Autodesk Fusion 360 part; units mm, degrees
(part 2 of 7)
  spline S30 degree 3 poles (-152.5, -27.3069) (-152.0881, -26.4817) (-151.6514, -25.2172) (-151.2668, -23.9183) (-150.7129, -22.0478) (-150.237, -20.0931) (-149.6002, -18.3797) (-148.9085, -16.5186) (-147.986, -14.8851) (-146.6355, -13.7409) (-146.4823, -13.6111) (-146.3242, -13.4878) (-146.1613, -13.3717) (-145.7742, -13.0956) (-145.3871, -12.8196) (-145, -12.5435) knots -0.398144 -0.398144 -0.398144 -0.398144 -0.30293 -0.30293 -0.30293 -0.165823 -0.165823 -0.165823 -0.016893 -0.016893 -0.016893 0 0 0 0.056001 0.056001 0.056001 0.056001
  spline S31 degree 3 poles (-145, -12.5435) (-144.6129, -12.8196) (-144.2258, -13.0956) (-143.8387, -13.3717) (-142.4048, -14.3943) (-141.3881, -15.9477) (-140.6468, -17.7479) (-139.9554, -19.4267) (-139.4675, -21.3627) (-138.9195, -23.2775) (-138.5808, -24.4611) (-138.2149, -25.6362) (-137.8326, -26.5675) (-137.7208, -26.8397) (-137.6088, -27.0889) (-137.5, -27.3069) knots -1.056001 -1.056001 -1.056001 -1.056001 -1 -1 -1 -0.851292 -0.851292 -0.851292 -0.71262 -0.71262 -0.71262 -0.626906 -0.626906 -0.626906 -0.601856 -0.601856 -0.601856 -0.601856
  spline S32 degree 3 poles (-137.5, -27.3069) (-137.0881, -26.4817) (-136.6514, -25.2172) (-136.2668, -23.9183) (-135.7129, -22.0478) (-135.237, -20.0931) (-134.6002, -18.3797) (-133.9085, -16.5186) (-132.986, -14.8851) (-131.6355, -13.7409) (-131.4823, -13.6111) (-131.3242, -13.4878) (-131.1613, -13.3717) (-130.7742, -13.0956) (-130.3871, -12.8196) (-130, -12.5435) knots -0.398144 -0.398144 -0.398144 -0.398144 -0.30293 -0.30293 -0.30293 -0.165823 -0.165823 -0.165823 -0.016893 -0.016893 -0.016893 0 0 0 0.056001 0.056001 0.056001 0.056001
  spline S33 degree 3 poles (-130, -12.5435) (-129.6129, -12.8196) (-129.2258, -13.0956) (-128.8387, -13.3717) (-127.4048, -14.3943) (-126.3881, -15.9477) (-125.6468, -17.7479) (-124.9554, -19.4267) (-124.4675, -21.3627) (-123.9195, -23.2775) (-123.5808, -24.4611) (-123.2149, -25.6362) (-122.8326, -26.5675) (-122.7208, -26.8397) (-122.6088, -27.0889) (-122.5, -27.3069) knots -1.056001 -1.056001 -1.056001 -1.056001 -1 -1 -1 -0.851292 -0.851292 -0.851292 -0.71262 -0.71262 -0.71262 -0.626906 -0.626906 -0.626906 -0.601856 -0.601856 -0.601856 -0.601856
  spline S34 degree 3 poles (-122.5, -27.3069) (-122.0881, -26.4817) (-121.6514, -25.2172) (-121.2668, -23.9183) (-120.7129, -22.0478) (-120.237, -20.0931) (-119.6002, -18.3797) (-118.9085, -16.5186) (-117.986, -14.8851) (-116.6355, -13.7409) (-116.4823, -13.6111) (-116.3242, -13.4878) (-116.1613, -13.3717) (-115.7742, -13.0956) (-115.3871, -12.8196) (-115, -12.5435) knots -0.398144 -0.398144 -0.398144 -0.398144 -0.30293 -0.30293 -0.30293 -0.165823 -0.165823 -0.165823 -0.016893 -0.016893 -0.016893 0 0 0 0.056001 0.056001 0.056001 0.056001
  spline S35 degree 3 poles (-115, -12.5435) (-114.6129, -12.8196) (-114.2258, -13.0956) (-113.8387, -13.3717) (-112.4048, -14.3943) (-111.3881, -15.9477) (-110.6468, -17.7479) (-109.9554, -19.4267) (-109.4675, -21.3627) (-108.9195, -23.2775) (-108.5808, -24.4611) (-108.2149, -25.6362) (-107.8326, -26.5675) (-107.7208, -26.8397) (-107.6088, -27.0889) (-107.5, -27.3069) knots -1.056001 -1.056001 -1.056001 -1.056001 -1 -1 -1 -0.851292 -0.851292 -0.851292 -0.71262 -0.71262 -0.71262 -0.626906 -0.626906 -0.626906 -0.601856 -0.601856 -0.601856 -0.601856
  spline S36 degree 3 poles (-107.5, -27.3069) (-107.0881, -26.4817) (-106.6514, -25.2172) (-106.2668, -23.9183) (-105.7129, -22.0478) (-105.237, -20.0931) (-104.6002, -18.3797) (-103.9085, -16.5186) (-102.986, -14.8851) (-101.6355, -13.7409) (-101.4823, -13.6111) (-101.3242, -13.4878) (-101.1613, -13.3717) (-100.7742, -13.0956) (-100.3871, -12.8196) (-100, -12.5435) knots -0.398144 -0.398144 -0.398144 -0.398144 -0.30293 -0.30293 -0.30293 -0.165823 -0.165823 -0.165823 -0.016893 -0.016893 -0.016893 0 0 0 0.056001 0.056001 0.056001 0.056001
  spline S37 degree 3 poles (-100, -12.5435) (-99.6129, -12.8196) (-99.2258, -13.0956) (-98.8387, -13.3717) (-97.4048, -14.3943) (-96.3881, -15.9477) (-95.6468, -17.7479) (-94.9554, -19.4267) (-94.4675, -21.3627) (-93.9195, -23.2775) (-93.5808, -24.4611) (-93.2149, -25.6362) (-92.8326, -26.5675) (-92.7208, -26.8397) (-92.6088, -27.0889) (-92.5, -27.3069) knots -1.056001 -1.056001 -1.056001 -1.056001 -1 -1 -1 -0.851292 -0.851292 -0.851292 -0.71262 -0.71262 -0.71262 -0.626906 -0.626906 -0.626906 -0.601856 -0.601856 -0.601856 -0.601856
  spline S38 degree 3 poles (-92.5, -27.3069) (-92.0881, -26.4817) (-91.6514, -25.2172) (-91.2668, -23.9183) (-90.7129, -22.0478) (-90.237, -20.0931) (-89.6002, -18.3797) (-88.9085, -16.5186) (-87.986, -14.8851) (-86.6355, -13.7409) (-86.4823, -13.6111) (-86.3242, -13.4878) (-86.1613, -13.3717) (-85.7742, -13.0956) (-85.3871, -12.8196) (-85, -12.5435) knots -0.398144 -0.398144 -0.398144 -0.398144 -0.30293 -0.30293 -0.30293 -0.165823 -0.165823 -0.165823 -0.016893 -0.016893 -0.016893 0 0 0 0.056001 0.056001 0.056001 0.056001
  spline S39 degree 3 poles (-85, -12.5435) (-84.6129, -12.8196) (-84.2258, -13.0956) (-83.8387, -13.3717) (-82.4048, -14.3943) (-81.3881, -15.9477) (-80.6468, -17.7479) (-79.9554, -19.4267) (-79.4675, -21.3627) (-78.9195, -23.2775) (-78.5808, -24.4611) (-78.2149, -25.6362) (-77.8326, -26.5675) (-77.7208, -26.8397) (-77.6088, -27.0889) (-77.5, -27.3069) knots -1.056001 -1.056001 -1.056001 -1.056001 -1 -1 -1 -0.851292 -0.851292 -0.851292 -0.71262 -0.71262 -0.71262 -0.626906 -0.626906 -0.626906 -0.601856 -0.601856 -0.601856 -0.601856
  spline S40 degree 3 poles (-77.5, -27.3069) (-77.0881, -26.4817) (-76.6514, -25.2172) (-76.2668, -23.9183) (-75.7129, -22.0478) (-75.237, -20.0931) (-74.6002, -18.3797) (-73.9085, -16.5186) (-72.986, -14.8851) (-71.6355, -13.7409) (-71.4823, -13.6111) (-71.3242, -13.4878) (-71.1613, -13.3717) (-70.7742, -13.0956) (-70.3871, -12.8196) (-70, -12.5435) knots -0.398144 -0.398144 -0.398144 -0.398144 -0.30293 -0.30293 -0.30293 -0.165823 -0.165823 -0.165823 -0.016893 -0.016893 -0.016893 0 0 0 0.056001 0.056001 0.056001 0.056001
  spline S41 degree 3 poles (-70, -12.5435) (-69.6129, -12.8196) (-69.2258, -13.0956) (-68.8387, -13.3717) (-67.4048, -14.3943) (-66.3881, -15.9477) (-65.6468, -17.7479) (-64.9554, -19.4267) (-64.4675, -21.3627) (-63.9195, -23.2775) (-63.5808, -24.4611) (-63.2149, -25.6362) (-62.8326, -26.5675) (-62.7208, -26.8397) (-62.6088, -27.0889) (-62.5, -27.3069) knots -1.056001 -1.056001 -1.056001 -1.056001 -1 -1 -1 -0.851292 -0.851292 -0.851292 -0.71262 -0.71262 -0.71262 -0.626906 -0.626906 -0.626906 -0.601856 -0.601856 -0.601856 -0.601856
  spline S42 degree 3 poles (-62.5, -27.3069) (-62.0881, -26.4817) (-61.6514, -25.2172) (-61.2668, -23.9183) (-60.7129, -22.0478) (-60.237, -20.0931) (-59.6002, -18.3797) (-58.9085, -16.5186) (-57.986, -14.8851) (-56.6355, -13.7409) (-56.4823, -13.6111) (-56.3242, -13.4878) (-56.1613, -13.3717) (-55.7742, -13.0956) (-55.3871, -12.8196) (-55, -12.5435) knots -0.398144 -0.398144 -0.398144 -0.398144 -0.30293 -0.30293 -0.30293 -0.165823 -0.165823 -0.165823 -0.016893 -0.016893 -0.016893 0 0 0 0.056001 0.056001 0.056001 0.056001
  spline S43 degree 3 poles (-55, -12.5435) (-54.6129, -12.8196) (-54.2258, -13.0956) (-53.8387, -13.3717) (-52.4048, -14.3943) (-51.3881, -15.9477) (-50.6468, -17.7479) (-49.9554, -19.4267) (-49.4675, -21.3627) (-48.9195, -23.2775) (-48.5808, -24.4611) (-48.2149, -25.6362) (-47.8326, -26.5675) (-47.7208, -26.8397) (-47.6088, -27.0889) (-47.5, -27.3069) knots -1.056001 -1.056001 -1.056001 -1.056001 -1 -1 -1 -0.851292 -0.851292 -0.851292 -0.71262 -0.71262 -0.71262 -0.626906 -0.626906 -0.626906 -0.601856 -0.601856 -0.601856 -0.601856
  spline S44 degree 3 poles (-47.5, -27.3069) (-47.0881, -26.4817) (-46.6514, -25.2172) (-46.2668, -23.9183) (-45.7129, -22.0478) (-45.237, -20.0931) (-44.6002, -18.3797) (-43.9085, -16.5186) (-42.986, -14.8851) (-41.6355, -13.7409) (-41.4823, -13.6111) (-41.3242, -13.4878) (-41.1613, -13.3717) (-40.7742, -13.0956) (-40.3871, -12.8196) (-40, -12.5435) knots -0.398144 -0.398144 -0.398144 -0.398144 -0.30293 -0.30293 -0.30293 -0.165823 -0.165823 -0.165823 -0.016893 -0.016893 -0.016893 0 0 0 0.056001 0.056001 0.056001 0.056001
  spline S45 degree 3 poles (-40, -12.5435) (-39.6129, -12.8196) (-39.2258, -13.0956) (-38.8387, -13.3717) (-37.4048, -14.3943) (-36.3881, -15.9477) (-35.6468, -17.7479) (-34.9554, -19.4267) (-34.4675, -21.3627) (-33.9195, -23.2775) (-33.5808, -24.4611) (-33.2149, -25.6362) (-32.8326, -26.5675) (-32.7208, -26.8397) (-32.6088, -27.0889) (-32.5, -27.3069) knots -1.056001 -1.056001 -1.056001 -1.056001 -1 -1 -1 -0.851292 -0.851292 -0.851292 -0.71262 -0.71262 -0.71262 -0.626906 -0.626906 -0.626906 -0.601856 -0.601856 -0.601856 -0.601856
  spline S46 degree 3 poles (-32.5, -27.3069) (-32.0881, -26.4817) (-31.6514, -25.2172) (-31.2668, -23.9183) (-30.7129, -22.0478) (-30.237, -20.0931) (-29.6002, -18.3797) (-28.9085, -16.5186) (-27.986, -14.8851) (-26.6355, -13.7409) (-26.4823, -13.6111) (-26.3242, -13.4878) (-26.1613, -13.3717) (-25.7742, -13.0956) (-25.3871, -12.8196) (-25, -12.5435) knots -0.398144 -0.398144 -0.398144 -0.398144 -0.30293 -0.30293 -0.30293 -0.165823 -0.165823 -0.165823 -0.016893 -0.016893 -0.016893 0 0 0 0.056001 0.056001 0.056001 0.056001
  arc A14 (-250, -12.5435) -> (-250, -3) centre (-250, -7.7718) ccw
  arc A15 (-25, -3) -> (-25, -12.5435) centre (-25, -7.7718) ccw
  constraint tangent L29 A14
  constraint coincident L29 A14.end
  constraint tangent L29 A15
  constraint coincident L29 A15.start
sketch "スケッチ6" plane through (0, 0, 2) normal (0, 0, 1) x (-1, 0, 0)
  spline S0 degree 3 poles (-242.5, -27.3069) (-242.6088, -27.0889) (-242.7208, -26.8397) (-242.8326, -26.5675) (-243.2149, -25.6362) (-243.5808, -24.4611) (-243.9195, -23.2775) (-244.4675, -21.3627) (-244.9554, -19.4267) (-245.6468, -17.7479) (-246.3881, -15.9477) (-247.4048, -14.3943) (-248.8387, -13.3717) (-249.2258, -13.0956) (-249.6129, -12.8196) (-250, -12.5435) knots 0.601856 0.601856 0.601856 0.601856 0.626906 0.626906 0.626906 0.71262 0.71262 0.71262 0.851292 0.851292 0.851292 1 1 1 1.056001 1.056001 1.056001 1.056001
  spline S1 degree 3 poles (-235, -12.5435) (-235.3871, -12.8196) (-235.7742, -13.0956) (-236.1613, -13.3717) (-236.3242, -13.4878) (-236.4823, -13.6111) (-236.6355, -13.7409) (-237.986, -14.8851) (-238.9085, -16.5186) (-239.6002, -18.3797) (-240.237, -20.0931) (-240.7129, -22.0478) (-241.2668, -23.9183) (-241.6514, -25.2172) (-242.0881, -26.4817) (-242.5, -27.3069) knots -0.056001 -0.056001 -0.056001 -0.056001 0 0 0 0.016893 0.016893 0.016893 0.165823 0.165823 0.165823 0.30293 0.30293 0.30293 0.398144 0.398144 0.398144 0.398144
  spline S2 degree 3 poles (-227.5, -27.3069) (-227.6088, -27.0889) (-227.7208, -26.8397) (-227.8326, -26.5675) (-228.2149, -25.6362) (-228.5808, -24.4611) (-228.9195, -23.2775) (-229.4675, -21.3627) (-229.9554, -19.4267) (-230.6468, -17.7479) (-231.3881, -15.9477) (-232.4048, -14.3943) (-233.8387, -13.3717) (-234.2258, -13.0956) (-234.6129, -12.8196) (-235, -12.5435) knots 0.601856 0.601856 0.601856 0.601856 0.626906 0.626906 0.626906 0.71262 0.71262 0.71262 0.851292 0.851292 0.851292 1 1 1 1.056001 1.056001 1.056001 1.056001
  spline S3 degree 3 poles (-220, -12.5435) (-220.3871, -12.8196) (-220.7742, -13.0956) (-221.1613, -13.3717) (-221.3242, -13.4878) (-221.4823, -13.6111) (-221.6355, -13.7409) (-222.986, -14.8851) (-223.9085, -16.5186) (-224.6002, -18.3797) (-225.237, -20.0931) (-225.7129, -22.0478) (-226.2668, -23.9183) (-226.6514, -25.2172) (-227.0881, -26.4817) (-227.5, -27.3069) knots -0.056001 -0.056001 -0.056001 -0.056001 0 0 0 0.016893 0.016893 0.016893 0.165823 0.165823 0.165823 0.30293 0.30293 0.30293 0.398144 0.398144 0.398144 0.398144
  spline S4 degree 3 poles (-212.5, -27.3069) (-212.6088, -27.0889) (-212.7208, -26.8397) (-212.8326, -26.5675) (-213.2149, -25.6362) (-213.5808, -24.4611) (-213.9195, -23.2775) (-214.4675, -21.3627) (-214.9554, -19.4267) (-215.6468, -17.7479) (-216.3881, -15.9477) (-217.4048, -14.3943) (-218.8387, -13.3717) (-219.2258, -13.0956) (-219.6129, -12.8196) (-220, -12.5435) knots 0.601856 0.601856 0.601856 0.601856 0.626906 0.626906 0.626906 0.71262 0.71262 0.71262 0.851292 0.851292 0.851292 1 1 1 1.056001 1.056001 1.056001 1.056001
  spline S5 degree 3 poles (-205, -12.5435) (-205.3871, -12.8196) (-205.7742, -13.0956) (-206.1613, -13.3717) (-206.3242, -13.4878) (-206.4823, -13.6111) (-206.6355, -13.7409) (-207.986, -14.8851) (-208.9085, -16.5186) (-209.6002, -18.3797) (-210.237, -20.0931) (-210.7129, -22.0478) (-211.2668, -23.9183) (-211.6514, -25.2172) (-212.0881, -26.4817) (-212.5, -27.3069) knots -0.056001 -0.056001 -0.056001 -0.056001 0 0 0 0.016893 0.016893 0.016893 0.165823 0.165823 0.165823 0.30293 0.30293 0.30293 0.398144 0.398144 0.398144 0.398144
  spline S6 degree 3 poles (-197.5, -27.3069) (-197.6088, -27.0889) (-197.7208, -26.8397) (-197.8326, -26.5675) (-198.2149, -25.6362) (-198.5808, -24.4611) (-198.9195, -23.2775) (-199.4675, -21.3627) (-199.9554, -19.4267) (-200.6468, -17.7479) (-201.3881, -15.9477) (-202.4048, -14.3943) (-203.8387, -13.3717) (-204.2258, -13.0956) (-204.6129, -12.8196) (-205, -12.5435) knots 0.601856 0.601856 0.601856 0.601856 0.626906 0.626906 0.626906 0.71262 0.71262 0.71262 0.851292 0.851292 0.851292 1 1 1 1.056001 1.056001 1.056001 1.056001
  spline S7 degree 3 poles (-190, -12.5435) (-190.3871, -12.8196) (-190.7742, -13.0956) (-191.1613, -13.3717) (-191.3242, -13.4878) (-191.4823, -13.6111) (-191.6355, -13.7409) (-192.986, -14.8851) (-193.9085, -16.5186) (-194.6002, -18.3797) (-195.237, -20.0931) (-195.7129, -22.0478) (-196.2668, -23.9183) (-196.6514, -25.2172) (-197.0881, -26.4817) (-197.5, -27.3069) knots -0.056001 -0.056001 -0.056001 -0.056001 0 0 0 0.016893 0.016893 0.016893 0.165823 0.165823 0.165823 0.30293 0.30293 0.30293 0.398144 0.398144 0.398144 0.398144
  spline S8 degree 3 poles (-182.5, -27.3069) (-182.6088, -27.0889) (-182.7208, -26.8397) (-182.8326, -26.5675) (-183.2149, -25.6362) (-183.5808, -24.4611) (-183.9195, -23.2775) (-184.4675, -21.3627) (-184.9554, -19.4267) (-185.6468, -17.7479) (-186.3881, -15.9477) (-187.4048, -14.3943) (-188.8387, -13.3717) (-189.2258, -13.0956) (-189.6129, -12.8196) (-190, -12.5435) knots 0.601856 0.601856 0.601856 0.601856 0.626906 0.626906 0.626906 0.71262 0.71262 0.71262 0.851292 0.851292 0.851292 1 1 1 1.056001 1.056001 1.056001 1.056001
  spline S9 degree 3 poles (-175, -12.5435) (-175.3871, -12.8196) (-175.7742, -13.0956) (-176.1613, -13.3717) (-176.3242, -13.4878) (-176.4823, -13.6111) (-176.6355, -13.7409) (-177.986, -14.8851) (-178.9085, -16.5186) (-179.6002, -18.3797) (-180.237, -20.0931) (-180.7129, -22.0478) (-181.2668, -23.9183) (-181.6514, -25.2172) (-182.0881, -26.4817) (-182.5, -27.3069) knots -0.056001 -0.056001 -0.056001 -0.056001 0 0 0 0.016893 0.016893 0.016893 0.165823 0.165823 0.165823 0.30293 0.30293 0.30293 0.398144 0.398144 0.398144 0.398144
  spline S10 degree 3 poles (-167.5, -27.3069) (-167.6088, -27.0889) (-167.7208, -26.8397) (-167.8326, -26.5675) (-168.2149, -25.6362) (-168.5808, -24.4611) (-168.9195, -23.2775) (-169.4675, -21.3627) (-169.9554, -19.4267) (-170.6468, -17.7479) (-171.3881, -15.9477) (-172.4048, -14.3943) (-173.8387, -13.3717) (-174.2258, -13.0956) (-174.6129, -12.8196) (-175, -12.5435) knots 0.601856 0.601856 0.601856 0.601856 0.626906 0.626906 0.626906 0.71262 0.71262 0.71262 0.851292 0.851292 0.851292 1 1 1 1.056001 1.056001 1.056001 1.056001
  spline S11 degree 3 poles (-160, -12.5435) (-160.3871, -12.8196) (-160.7742, -13.0956) (-161.1613, -13.3717) (-161.3242, -13.4878) (-161.4823, -13.6111) (-161.6355, -13.7409) (-162.986, -14.8851) (-163.9085, -16.5186) (-164.6002, -18.3797) (-165.237, -20.0931) (-165.7129, -22.0478) (-166.2668, -23.9183) (-166.6514, -25.2172) (-167.0881, -26.4817) (-167.5, -27.3069) knots -0.056001 -0.056001 -0.056001 -0.056001 0 0 0 0.016893 0.016893 0.016893 0.165823 0.165823 0.165823 0.30293 0.30293 0.30293 0.398144 0.398144 0.398144 0.398144
  spline S12 degree 3 poles (-152.5, -27.3069) (-152.6088, -27.0889) (-152.7208, -26.8397) (-152.8326, -26.5675) (-153.2149, -25.6362) (-153.5808, -24.4611) (-153.9195, -23.2775) (-154.4675, -21.3627) (-154.9554, -19.4267) (-155.6468, -17.7479) (-156.3881, -15.9477) (-157.4048, -14.3943) (-158.8387, -13.3717) (-159.2258, -13.0956) (-159.6129, -12.8196) (-160, -12.5435) knots 0.601856 0.601856 0.601856 0.601856 0.626906 0.626906 0.626906 0.71262 0.71262 0.71262 0.851292 0.851292 0.851292 1 1 1 1.056001 1.056001 1.056001 1.056001
  spline S13 degree 3 poles (-145, -12.5435) (-145.3871, -12.8196) (-145.7742, -13.0956) (-146.1613, -13.3717) (-146.3242, -13.4878) (-146.4823, -13.6111) (-146.6355, -13.7409) (-147.986, -14.8851) (-148.9085, -16.5186) (-149.6002, -18.3797) (-150.237, -20.0931) (-150.7129, -22.0478) (-151.2668, -23.9183) (-151.6514, -25.2172) (-152.0881, -26.4817) (-152.5, -27.3069) knots -0.056001 -0.056001 -0.056001 -0.056001 0 0 0 0.016893 0.016893 0.016893 0.165823 0.165823 0.165823 0.30293 0.30293 0.30293 0.398144 0.398144 0.398144 0.398144
  spline S14 degree 3 poles (-137.5, -27.3069) (-137.6088, -27.0889) (-137.7208, -26.8397) (-137.8326, -26.5675) (-138.2149, -25.6362) (-138.5808, -24.4611) (-138.9195, -23.2775) (-139.4675, -21.3627) (-139.9554, -19.4267) (-140.6468, -17.7479) (-141.3881, -15.9477) (-142.4048, -14.3943) (-143.8387, -13.3717) (-144.2258, -13.0956) (-144.6129, -12.8196) (-145, -12.5435) knots 0.601856 0.601856 0.601856 0.601856 0.626906 0.626906 0.626906 0.71262 0.71262 0.71262 0.851292 0.851292 0.851292 1 1 1 1.056001 1.056001 1.056001 1.056001
  spline S15 degree 3 poles (-130, -12.5435) (-130.3871, -12.8196) (-130.7742, -13.0956) (-131.1613, -13.3717) (-131.3242, -13.4878) (-131.4823, -13.6111) (-131.6355, -13.7409) (-132.986, -14.8851) (-133.9085, -16.5186) (-134.6002, -18.3797) (-135.237, -20.0931) (-135.7129, -22.0478) (-136.2668, -23.9183) (-136.6514, -25.2172) (-137.0881, -26.4817) (-137.5, -27.3069) knots -0.056001 -0.056001 -0.056001 -0.056001 0 0 0 0.016893 0.016893 0.016893 0.165823 0.165823 0.165823 0.30293 0.30293 0.30293 0.398144 0.398144 0.398144 0.398144
  spline S16 degree 3 poles (-122.5, -27.3069) (-122.6088, -27.0889) (-122.7208, -26.8397) (-122.8326, -26.5675) (-123.2149, -25.6362) (-123.5808, -24.4611) (-123.9195, -23.2775) (-124.4675, -21.3627) (-124.9554, -19.4267) (-125.6468, -17.7479) (-126.3881, -15.9477) (-127.4048, -14.3943) (-128.8387, -13.3717) (-129.2258, -13.0956) (-129.6129, -12.8196) (-130, -12.5435) knots 0.601856 0.601856 0.601856 0.601856 0.626906 0.626906 0.626906 0.71262 0.71262 0.71262 0.851292 0.851292 0.851292 1 1 1 1.056001 1.056001 1.056001 1.056001
  spline S17 degree 3 poles (-115, -12.5435) (-115.3871, -12.8196) (-115.7742, -13.0956) (-116.1613, -13.3717) (-116.3242, -13.4878) (-116.4823, -13.6111) (-116.6355, -13.7409) (-117.986, -14.8851) (-118.9085, -16.5186) (-119.6002, -18.3797) (-120.237, -20.0931) (-120.7129, -22.0478) (-121.2668, -23.9183) (-121.6514, -25.2172) (-122.0881, -26.4817) (-122.5, -27.3069) knots -0.056001 -0.056001 -0.056001 -0.056001 0 0 0 0.016893 0.016893 0.016893 0.165823 0.165823 0.165823 0.30293 0.30293 0.30293 0.398144 0.398144 0.398144 0.398144
  spline S18 degree 3 poles (-107.5, -27.3069) (-107.6088, -27.0889) (-107.7208, -26.8397) (-107.8326, -26.5675) (-108.2149, -25.6362) (-108.5808, -24.4611) (-108.9195, -23.2775) (-109.4675, -21.3627) (-109.9554, -19.4267) (-110.6468, -17.7479) (-111.3881, -15.9477) (-112.4048, -14.3943) (-113.8387, -13.3717) (-114.2258, -13.0956) (-114.6129, -12.8196) (-115, -12.5435) knots 0.601856 0.601856 0.601856 0.601856 0.626906 0.626906 0.626906 0.71262 0.71262 0.71262 0.851292 0.851292 0.851292 1 1 1 1.056001 1.056001 1.056001 1.056001
  spline S19 degree 3 poles (-100, -12.5435) (-100.3871, -12.8196) (-100.7742, -13.0956) (-101.1613, -13.3717) (-101.3242, -13.4878) (-101.4823, -13.6111) (-101.6355, -13.7409) (-102.986, -14.8851) (-103.9085, -16.5186) (-104.6002, -18.3797) (-105.237, -20.0931) (-105.7129, -22.0478) (-106.2668, -23.9183) (-106.6514, -25.2172) (-107.0881, -26.4817) (-107.5, -27.3069) knots -0.056001 -0.056001 -0.056001 -0.056001 0 0 0 0.016893 0.016893 0.016893 0.165823 0.165823 0.165823 0.30293 0.30293 0.30293 0.398144 0.398144 0.398144 0.398144
  spline S20 degree 3 poles (-92.5, -27.3069) (-92.6088, -27.0889) (-92.7208, -26.8397) (-92.8326, -26.5675) (-93.2149, -25.6362) (-93.5808, -24.4611) (-93.9195, -23.2775) (-94.4675, -21.3627) (-94.9554, -19.4267) (-95.6468, -17.7479) (-96.3881, -15.9477) (-97.4048, -14.3943) (-98.8387, -13.3717) (-99.2258, -13.0956) (-99.6129, -12.8196) (-100, -12.5435) knots 0.601856 0.601856 0.601856 0.601856 0.626906 0.626906 0.626906 0.71262 0.71262 0.71262 0.851292 0.851292 0.851292 1 1 1 1.056001 1.056001 1.056001 1.056001
  spline S21 degree 3 poles (-85, -12.5435) (-85.3871, -12.8196) (-85.7742, -13.0956) (-86.1613, -13.3717) (-86.3242, -13.4878) (-86.4823, -13.6111) (-86.6355, -13.7409) (-87.986, -14.8851) (-88.9085, -16.5186) (-89.6002, -18.3797) (-90.237, -20.0931) (-90.7129, -22.0478) (-91.2668, -23.9183) (-91.6514, -25.2172) (-92.0881, -26.4817) (-92.5, -27.3069) knots -0.056001 -0.056001 -0.056001 -0.056001 0 0 0 0.016893 0.016893 0.016893 0.165823 0.165823 0.165823 0.30293 0.30293 0.30293 0.398144 0.398144 0.398144 0.398144
  spline S22 degree 3 poles (-77.5, -27.3069) (-77.6088, -27.0889) (-77.7208, -26.8397) (-77.8326, -26.5675) (-78.2149, -25.6362) (-78.5808, -24.4611) (-78.9195, -23.2775) (-79.4675, -21.3627) (-79.9554, -19.4267) (-80.6468, -17.7479) (-81.3881, -15.9477) (-82.4048, -14.3943) (-83.8387, -13.3717) (-84.2258, -13.0956) (-84.6129, -12.8196) (-85, -12.5435) knots 0.601856 0.601856 0.601856 0.601856 0.626906 0.626906 0.626906 0.71262 0.71262 0.71262 0.851292 0.851292 0.851292 1 1 1 1.056001 1.056001 1.056001 1.056001
  spline S23 degree 3 poles (-70, -12.5435) (-70.3871, -12.8196) (-70.7742, -13.0956) (-71.1613, -13.3717) (-71.3242, -13.4878) (-71.4823, -13.6111) (-71.6355, -13.7409) (-72.986, -14.8851) (-73.9085, -16.5186) (-74.6002, -18.3797) (-75.237, -20.0931) (-75.7129, -22.0478) (-76.2668, -23.9183) (-76.6514, -25.2172) (-77.0881, -26.4817) (-77.5, -27.3069) knots -0.056001 -0.056001 -0.056001 -0.056001 0 0 0 0.016893 0.016893 0.016893 0.165823 0.165823 0.165823 0.30293 0.30293 0.30293 0.398144 0.398144 0.398144 0.398144
  spline S24 degree 3 poles (-62.5, -27.3069) (-62.6088, -27.0889) (-62.7208, -26.8397) (-62.8326, -26.5675) (-63.2149, -25.6362) (-63.5808, -24.4611) (-63.9195, -23.2775) (-64.4675, -21.3627) (-64.9554, -19.4267) (-65.6468, -17.7479) (-66.3881, -15.9477) (-67.4048, -14.3943) (-68.8387, -13.3717) (-69.2258, -13.0956) (-69.6129, -12.8196) (-70, -12.5435) knots 0.601856 0.601856 0.601856 0.601856 0.626906 0.626906 0.626906 0.71262 0.71262 0.71262 0.851292 0.851292 0.851292 1 1 1 1.056001 1.056001 1.056001 1.056001
  spline S25 degree 3 poles (-55, -12.5435) (-55.3871, -12.8196) (-55.7742, -13.0956) (-56.1613, -13.3717) (-56.3242, -13.4878) (-56.4823, -13.6111) (-56.6355, -13.7409) (-57.986, -14.8851) (-58.9085, -16.5186) (-59.6002, -18.3797) (-60.237, -20.0931) (-60.7129, -22.0478) (-61.2668, -23.9183) (-61.6514, -25.2172) (-62.0881, -26.4817) (-62.5, -27.3069) knots -0.056001 -0.056001 -0.056001 -0.056001 0 0 0 0.016893 0.016893 0.016893 0.165823 0.165823 0.165823 0.30293 0.30293 0.30293 0.398144 0.398144 0.398144 0.398144
  spline S26 degree 3 poles (-47.5, -27.3069) (-47.6088, -27.0889) (-47.7208, -26.8397) (-47.8326, -26.5675) (-48.2149, -25.6362) (-48.5808, -24.4611) (-48.9195, -23.2775) (-49.4675, -21.3627) (-49.9554, -19.4267) (-50.6468, -17.7479) (-51.3881, -15.9477) (-52.4048, -14.3943) (-53.8387, -13.3717) (-54.2258, -13.0956) (-54.6129, -12.8196) (-55, -12.5435) knots 0.601856 0.601856 0.601856 0.601856 0.626906 0.626906 0.626906 0.71262 0.71262 0.71262 0.851292 0.851292 0.851292 1 1 1 1.056001 1.056001 1.056001 1.056001
  spline S27 degree 3 poles (-40, -12.5435) (-40.3871, -12.8196) (-40.7742, -13.0956) (-41.1613, -13.3717) (-41.3242, -13.4878) (-41.4823, -13.6111) (-41.6355, -13.7409) (-42.986, -14.8851) (-43.9085, -16.5186) (-44.6002, -18.3797) (-45.237, -20.0931) (-45.7129, -22.0478) (-46.2668, -23.9183) (-46.6514, -25.2172) (-47.0881, -26.4817) (-47.5, -27.3069) knots -0.056001 -0.056001 -0.056001 -0.056001 0 0 0 0.016893 0.016893 0.016893 0.165823 0.165823 0.165823 0.30293 0.30293 0.30293 0.398144 0.398144 0.398144 0.398144
  spline S28 degree 3 poles (-32.5, -27.3069) (-32.6088, -27.0889) (-32.7208, -26.8397) (-32.8326, -26.5675) (-33.2149, -25.6362) (-33.5808, -24.4611) (-33.9195, -23.2775) (-34.4675, -21.3627) (-34.9554, -19.4267) (-35.6468, -17.7479) (-36.3881, -15.9477) (-37.4048, -14.3943) (-38.8387, -13.3717) (-39.2258, -13.0956) (-39.6129, -12.8196) (-40, -12.5435) knots 0.601856 0.601856 0.601856 0.601856 0.626906 0.626906 0.626906 0.71262 0.71262 0.71262 0.851292 0.851292 0.851292 1 1 1 1.056001 1.056001 1.056001 1.056001
  spline S29 degree 3 poles (-25, -12.5435) (-25.3871, -12.8196) (-25.7742, -13.0956) (-26.1613, -13.3717) (-26.3242, -13.4878) (-26.4823, -13.6111) (-26.6355, -13.7409) (-27.986, -14.8851) (-28.9085, -16.5186) (-29.6002, -18.3797) (-30.237, -20.0931) (-30.7129, -22.0478) (-31.2668, -23.9183) (-31.6514, -25.2172) (-32.0881, -26.4817) (-32.5, -27.3069) knots -0.056001 -0.056001 -0.056001 -0.056001 0 0 0 0.016893 0.016893 0.016893 0.165823 0.165823 0.165823 0.30293 0.30293 0.30293 0.398144 0.398144 0.398144 0.398144
  arc A0 (-25, -3) -> (-25, -12.5435) centre (-25, -7.7718) ccw
  line L0 (-25, -3) -> (-250, -3)
  arc A1 (-250, -12.5435) -> (-250, -3) centre (-250, -7.7718) ccw
  line L1 (-32.0304, -4.4213) -> (-39.033, -9.3231)
  line L2 (-41.5, -10) -> (-232, -10)
  line L3 (-236.5484, -8.9161) -> (-242.5709, -4.7004)
  arc A2 (-242.5709, -4.7004) -> (-247.5, -3) centre (-248.0084, -12.4682) ccw
  arc A3 (-28.5, -3) -> (-32.0304, -4.4213) centre (-27.2024, -11.3185) ccw
  arc A4 (-41.5, -10) -> (-38.4384, -8.9069) centre (-41.5, -5.166) ccw
  arc A5 (-236.5484, -8.9161) -> (-232, -10) centre (-232, 0.0854) ccw
  constraint parallel L0 L2
  constraint tangent L3 A2
  constraint coincident L0 A2.end
  constraint tangent L1 A3
  constraint coincident L0 A3.start
  constraint tangent L2 A4
  constraint coincident L1 A4.end
  constraint coincident A4 L1.end
  constraint tangent L2 A5
sketch "スケッチ7" plane through (0, 0, 0) normal (0, 0, 1) x (1, 0, 0)
  spline S0 degree 5 poles (70, -85) (70.1382, -84.9014) (70.4088, -84.691) (70.7966, -84.3357) (71.2779, -83.7824) (71.8206, -82.9585) (72.3075, -82.0039) (72.7453, -80.9239) (73.1463, -79.7274) (73.5274, -78.4298) (73.9072, -77.0547) (74.3043, -75.6366) (74.7345, -74.223) (75.2088, -72.8764) (75.7302, -71.6789) (76.2937, -70.7262) (76.8886, -70.1082) (77.5, -69.8927) (78.1114, -70.1082) (78.7063, -70.7262) (79.2698, -71.6789) (79.7912, -72.8764) (80.2655, -74.223) (80.6957, -75.6366) (81.0928, -77.0547) (81.4726, -78.4298) (81.8537, -79.7274) (82.2547, -80.9239) (82.6925, -82.0039) (83.1794, -82.9585) (83.7221, -83.7824) (84.2034, -84.3357) (84.5912, -84.691) (84.8618, -84.9014) (85, -85) knots 0 0 0 0 0 0 0.033333 0.066667 0.1 0.133333 0.166667 0.2 0.233333 0.266667 0.3 0.333333 0.366667 0.4 0.433333 0.466667 0.5 0.533333 0.566667 0.6 0.633333 0.666667 0.7 0.733333 0.766667 0.8 0.833333 0.866667 0.9 0.933333 0.966667 1 1 1 1 1 1
  arc A0 (22, -90.4891) -> (22, -89.508) centre (22.0093, -89.9985) ccw
  line L0 (7.5, -91.5) -> (3, -91.5)
  arc A1 (22, -92.5) -> (22, -91.5) centre (22, -92) ccw
  line L1 (257.0187, -89.508) -> (250.0532, -89.508)
  spline S1 degree 5 poles (25, -85) (25.1382, -84.9014) (25.4088, -84.691) (25.7966, -84.3357) (26.2779, -83.7824) (26.8206, -82.9585) (27.3075, -82.0039) (27.7453, -80.9239) (28.1463, -79.7274) (28.5274, -78.4298) (28.9072, -77.0547) (29.3043, -75.6366) (29.7345, -74.223) (30.2088, -72.8764) (30.7302, -71.6789) (31.2937, -70.7262) (31.8886, -70.1082) (32.5, -69.8927) (33.1114, -70.1082) (33.7063, -70.7262) (34.2698, -71.6789) (34.7912, -72.8764) (35.2655, -74.223) (35.6957, -75.6366) (36.0928, -77.0547) (36.4726, -78.4298) (36.8537, -79.7274) (37.2547, -80.9239) (37.6925, -82.0039) (38.1794, -82.9585) (38.7221, -83.7824) (39.2034, -84.3357) (39.5912, -84.691) (39.8618, -84.9014) (40, -85) knots 0 0 0 0 0 0 0.033333 0.066667 0.1 0.133333 0.166667 0.2 0.233333 0.266667 0.3 0.333333 0.366667 0.4 0.433333 0.466667 0.5 0.533333 0.566667 0.6 0.633333 0.666667 0.7 0.733333 0.766667 0.8 0.833333 0.866667 0.9 0.933333 0.966667 1 1 1 1 1 1
  line L2 (5.5, -97) -> (254.5, -97)
  line L3 (252.5, -91.5) -> (250, -94)
  line L4 (22.0187, -89.508) -> (15.0532, -89.508)
  line L5 (245, -95) -> (250, -95)
  arc A2 (238, -89.508) -> (238, -90.4891) centre (237.9907, -89.9985) ccw
  arc A3 (250.0532, -89.508) -> (244.9467, -89.508) centre (247.5, -89.9985) ccw
  spline S2 degree 5 poles (205, -85) (205.1382, -84.9014) (205.4088, -84.691) (205.7966, -84.3357) (206.2779, -83.7824) (206.8206, -82.9585) (207.3075, -82.0039) (207.7453, -80.9239) (208.1463, -79.7274) (208.5274, -78.4298) (208.9072, -77.0547) (209.3043, -75.6366) (209.7345, -74.223) (210.2088, -72.8764) (210.7302, -71.6789) (211.2937, -70.7262) (211.8886, -70.1082) (212.5, -69.8927) (213.1114, -70.1082) (213.7063, -70.7262) (214.2698, -71.6789) (214.7912, -72.8764) (215.2655, -74.223) (215.6957, -75.6366) (216.0928, -77.0547) (216.4726, -78.4298) (216.8537, -79.7274) (217.2547, -80.9239) (217.6925, -82.0039) (218.1794, -82.9585) (218.7221, -83.7824) (219.2034, -84.3357) (219.5912, -84.691) (219.8618, -84.9014) (220, -85) knots 0 0 0 0 0 0 0.033333 0.066667 0.1 0.133333 0.166667 0.2 0.233333 0.266667 0.3 0.333333 0.366667 0.4 0.433333 0.466667 0.5 0.533333 0.566667 0.6 0.633333 0.666667 0.7 0.733333 0.766667 0.8 0.833333 0.866667 0.9 0.933333 0.966667 1 1 1 1 1 1
  line L6 (10, -95) -> (15, -95)
  line L7 (2.9813, -90.4891) -> (9.9466, -90.4891)
  line L8 (15, -95) -> (17.5, -92.5)
  line L9 (3, -92.5) -> (7.5, -92.5)
  spline S3 degree 5 poles (40, -85) (40.1382, -84.9014) (40.4088, -84.691) (40.7966, -84.3357) (41.2779, -83.7824) (41.8206, -82.9585) (42.3075, -82.0039) (42.7453, -80.9239) (43.1463, -79.7274) (43.5274, -78.4298) (43.9072, -77.0547) (44.3043, -75.6366) (44.7345, -74.223) (45.2088, -72.8764) (45.7302, -71.6789) (46.2937, -70.7262) (46.8886, -70.1082) (47.5, -69.8927) (48.1114, -70.1082) (48.7063, -70.7262) (49.2698, -71.6789) (49.7912, -72.8764) (50.2655, -74.223) (50.6957, -75.6366) (51.0928, -77.0547) (51.4726, -78.4298) (51.8537, -79.7274) (52.2547, -80.9239) (52.6925, -82.0039) (53.1794, -82.9585) (53.7221, -83.7824) (54.2034, -84.3357) (54.5912, -84.691) (54.8618, -84.9014) (55, -85) knots 0 0 0 0 0 0 0.033333 0.066667 0.1 0.133333 0.166667 0.2 0.233333 0.266667 0.3 0.333333 0.366667 0.4 0.433333 0.466667 0.5 0.533333 0.566667 0.6 0.633333 0.666667 0.7 0.733333 0.766667 0.8 0.833333 0.866667 0.9 0.933333 0.966667 1 1 1 1 1 1
  spline S4 degree 5 poles (10, -85) (10.1382, -84.9014) (10.4088, -84.691) (10.7966, -84.3357) (11.2779, -83.7824) (11.8206, -82.9585) (12.3075, -82.0039) (12.7453, -80.9239) (13.1463, -79.7274) (13.5274, -78.4298) (13.9072, -77.0547) (14.3043, -75.6366) (14.7345, -74.223) (15.2088, -72.8764) (15.7302, -71.6789) (16.2937, -70.7262) (16.8886, -70.1082) (17.5, -69.8927) (18.1114, -70.1082) (18.7063, -70.7262) (19.2698, -71.6789) (19.7912, -72.8764) (20.2655, -74.223) (20.6957, -75.6366) (21.0928, -77.0547) (21.4726, -78.4298) (21.8537, -79.7274) (22.2547, -80.9239) (22.6925, -82.0039) (23.1794, -82.9585) (23.7221, -83.7824) (24.2034, -84.3357) (24.5912, -84.691) (24.8618, -84.9014) (25, -85) knots 0 0 0 0 0 0 0.033333 0.066667 0.1 0.133333 0.166667 0.2 0.233333 0.266667 0.3 0.333333 0.366667 0.4 0.433333 0.466667 0.5 0.533333 0.566667 0.6 0.633333 0.666667 0.7 0.733333 0.766667 0.8 0.833333 0.866667 0.9 0.933333 0.966667 1 1 1 1 1 1
  spline S5 degree 5 poles (220, -85) (220.1382, -84.9014) (220.4088, -84.691) (220.7966, -84.3357) (221.2779, -83.7824) (221.8206, -82.9585) (222.3075, -82.0039) (222.7453, -80.9239) (223.1463, -79.7274) (223.5274, -78.4298) (223.9072, -77.0547) (224.3043, -75.6366) (224.7345, -74.223) (225.2088, -72.8764) (225.7302, -71.6789) (226.2937, -70.7262) (226.8886, -70.1082) (227.5, -69.8927) (228.1114, -70.1082) (228.7063, -70.7262) (229.2698, -71.6789) (229.7912, -72.8764) (230.2655, -74.223) (230.6957, -75.6366) (231.0928, -77.0547) (231.4726, -78.4298) (231.8537, -79.7274) (232.2547, -80.9239) (232.6925, -82.0039) (233.1794, -82.9585) (233.7221, -83.7824) (234.2034, -84.3357) (234.5912, -84.691) (234.8618, -84.9014) (235, -85) knots 0 0 0 0 0 0 0.033333 0.066667 0.1 0.133333 0.166667 0.2 0.233333 0.266667 0.3 0.333333 0.366667 0.4 0.433333 0.466667 0.5 0.533333 0.566667 0.6 0.633333 0.666667 0.7 0.733333 0.766667 0.8 0.833333 0.866667 0.9 0.933333 0.966667 1 1 1 1 1 1
  spline S6 degree 5 poles (85, -85) (85.1382, -84.9014) (85.4088, -84.691) (85.7966, -84.3357) (86.2779, -83.7824) (86.8206, -82.9585) (87.3075, -82.0039) (87.7453, -80.9239) (88.1463, -79.7274) (88.5274, -78.4298) (88.9072, -77.0547) (89.3043, -75.6366) (89.7345, -74.223) (90.2088, -72.8764) (90.7302, -71.6789) (91.2937, -70.7262) (91.8886, -70.1082) (92.5, -69.8927) (93.1114, -70.1082) (93.7063, -70.7262) (94.2698, -71.6789) (94.7912, -72.8764) (95.2655, -74.223) (95.6957, -75.6366) (96.0928, -77.0547) (96.4726, -78.4298) (96.8537, -79.7274) (97.2547, -80.9239) (97.6925, -82.0039) (98.1794, -82.9585) (98.7221, -83.7824) (99.2034, -84.3357) (99.5912, -84.691) (99.8618, -84.9014) (100, -85) knots 0 0 0 0 0 0 0.033333 0.066667 0.1 0.133333 0.166667 0.2 0.233333 0.266667 0.3 0.333333 0.366667 0.4 0.433333 0.466667 0.5 0.533333 0.566667 0.6 0.633333 0.666667 0.7 0.733333 0.766667 0.8 0.833333 0.866667 0.9 0.933333 0.966667 1 1 1 1 1 1
  line L10 (17.5, -91.5) -> (15, -94)
  spline S7 degree 5 poles (55, -85) (55.1382, -84.9014) (55.4088, -84.691) (55.7966, -84.3357) (56.2779, -83.7824) (56.8206, -82.9585) (57.3075, -82.0039) (57.7453, -80.9239) (58.1463, -79.7274) (58.5274, -78.4298) (58.9072, -77.0547) (59.3043, -75.6366) (59.7345, -74.223) (60.2088, -72.8764) (60.7302, -71.6789) (61.2937, -70.7262) (61.8886, -70.1082) (62.5, -69.8927) (63.1114, -70.1082) (63.7063, -70.7262) (64.2698, -71.6789) (64.7912, -72.8764) (65.2655, -74.223) (65.6957, -75.6366) (66.0928, -77.0547) (66.4726, -78.4298) (66.8537, -79.7274) (67.2547, -80.9239) (67.6925, -82.0039) (68.1794, -82.9585) (68.7221, -83.7824) (69.2034, -84.3357) (69.5912, -84.691) (69.8618, -84.9014) (70, -85) knots 0 0 0 0 0 0 0.033333 0.066667 0.1 0.133333 0.166667 0.2 0.233333 0.266667 0.3 0.333333 0.366667 0.4 0.433333 0.466667 0.5 0.533333 0.566667 0.6 0.633333 0.666667 0.7 0.733333 0.766667 0.8 0.833333 0.866667 0.9 0.933333 0.966667 1 1 1 1 1 1
  spline S8 degree 5 poles (235, -85) (235.1382, -84.9014) (235.4088, -84.691) (235.7966, -84.3357) (236.2779, -83.7824) (236.8206, -82.9585) (237.3075, -82.0039) (237.7453, -80.9239) (238.1463, -79.7274) (238.5274, -78.4298) (238.9072, -77.0547) (239.3043, -75.6366) (239.7345, -74.223) (240.2088, -72.8764) (240.7302, -71.6789) (241.2937, -70.7262) (241.8886, -70.1082) (242.5, -69.8927) (243.1114, -70.1082) (243.7063, -70.7262) (244.2698, -71.6789) (244.7912, -72.8764) (245.2655, -74.223) (245.6957, -75.6366) (246.0928, -77.0547) (246.4726, -78.4298) (246.8537, -79.7274) (247.2547, -80.9239) (247.6925, -82.0039) (248.1794, -82.9585) (248.7221, -83.7824) (249.2034, -84.3357) (249.5912, -84.691) (249.8618, -84.9014) (250, -85) knots 0 0 0 0 0 0 0.033333 0.066667 0.1 0.133333 0.166667 0.2 0.233333 0.266667 0.3 0.333333 0.366667 0.4 0.433333 0.466667 0.5 0.533333 0.566667 0.6 0.633333 0.666667 0.7 0.733333 0.766667 0.8 0.833333 0.866667 0.9 0.933333 0.966667 1 1 1 1 1 1
  line L11 (245, -94) -> (242.5, -91.5)
  arc A4 (3, -89.508) -> (3, -90.4891) centre (2.9907, -89.9985) ccw
  spline S9 degree 5 poles (190, -85) (190.1382, -84.9014) (190.4088, -84.691) (190.7966, -84.3357) (191.2779, -83.7824) (191.8206, -82.9585) (192.3075, -82.0039) (192.7453, -80.9239) (193.1463, -79.7274) (193.5274, -78.4298) (193.9072, -77.0547) (194.3043, -75.6366) (194.7345, -74.223) (195.2088, -72.8764) (195.7302, -71.6789) (196.2937, -70.7262) (196.8886, -70.1082) (197.5, -69.8927) (198.1114, -70.1082) (198.7063, -70.7262) (199.2698, -71.6789) (199.7912, -72.8764) (200.2655, -74.223) (200.6957, -75.6366) (201.0928, -77.0547) (201.4726, -78.4298) (201.8537, -79.7274) (202.2547, -80.9239) (202.6925, -82.0039) (203.1794, -82.9585) (203.7221, -83.7824) (204.2034, -84.3357) (204.5912, -84.691) (204.8618, -84.9014) (205, -85) knots 0 0 0 0 0 0 0.033333 0.066667 0.1 0.133333 0.166667 0.2 0.233333 0.266667 0.3 0.333333 0.366667 0.4 0.433333 0.466667 0.5 0.533333 0.566667 0.6 0.633333 0.666667 0.7 0.733333 0.766667 0.8 0.833333 0.866667 0.9 0.933333 0.966667 1 1 1 1 1 1
  arc A5 (3, -91.5) -> (3, -92.5) centre (3, -92) ccw
  line L12 (15, -94) -> (10, -94)
  line L13 (15.0533, -90.4891) -> (22.0187, -90.4891)
  arc A6 (257, -92.5) -> (257, -91.5) centre (257, -92) ccw
  line L14 (22, -91.5) -> (17.5, -91.5)
  arc A7 (257, -90.4891) -> (257, -89.508) centre (257.0093, -89.9985) ccw
  line L15 (7.5, -92.5) -> (10, -95)
  line L16 (10, -94) -> (7.5, -91.5)
  line L17 (237.9813, -90.4891) -> (244.9466, -90.4891)
  spline S10 degree 5 poles (115, -85) (115.1382, -84.9014) (115.4088, -84.691) (115.7966, -84.3357) (116.2779, -83.7824) (116.8206, -82.9585) (117.3075, -82.0039) (117.7453, -80.9239) (118.1463, -79.7274) (118.5274, -78.4298) (118.9072, -77.0547) (119.3043, -75.6366) (119.7345, -74.223) (120.2088, -72.8764) (120.7302, -71.6789) (121.2937, -70.7262) (121.8886, -70.1082) (122.5, -69.8927) (123.1114, -70.1082) (123.7063, -70.7262) (124.2698, -71.6789) (124.7912, -72.8764) (125.2655, -74.223) (125.6957, -75.6366) (126.0928, -77.0547) (126.4726, -78.4298) (126.8537, -79.7274) (127.2547, -80.9239) (127.6925, -82.0039) (128.1794, -82.9585) (128.7221, -83.7824) (129.2034, -84.3357) (129.5912, -84.691) (129.8618, -84.9014) (130, -85) knots 0 0 0 0 0 0 0.033333 0.066667 0.1 0.133333 0.166667 0.2 0.233333 0.266667 0.3 0.333333 0.366667 0.4 0.433333 0.466667 0.5 0.533333 0.566667 0.6 0.633333 0.666667 0.7 0.733333 0.766667 0.8 0.833333 0.866667 0.9 0.933333 0.966667 1 1 1 1 1 1
  line L18 (257, -91.5) -> (252.5, -91.5)
  line L19 (250, -94) -> (245, -94)
  arc A8 (15.0532, -89.508) -> (9.9467, -89.508) centre (12.5, -89.9985) ccw
  arc A9 (254.5, -97) -> (260.1618, -89.0141) centre (254.5, -91) ccw
  line L20 (242.5, -92.5) -> (245, -95)
  spline S11 degree 5 poles (145, -85) (145.1382, -84.9014) (145.4088, -84.691) (145.7966, -84.3357) (146.2779, -83.7824) (146.8206, -82.9585) (147.3075, -82.0039) (147.7453, -80.9239) (148.1463, -79.7274) (148.5274, -78.4298) (148.9072, -77.0547) (149.3043, -75.6366) (149.7345, -74.223) (150.2088, -72.8764) (150.7302, -71.6789) (151.2937, -70.7262) (151.8886, -70.1082) (152.5, -69.8927) (153.1114, -70.1082) (153.7063, -70.7262) (154.2698, -71.6789) (154.7912, -72.8764) (155.2655, -74.223) (155.6957, -75.6366) (156.0928, -77.0547) (156.4726, -78.4298) (156.8537, -79.7274) (157.2547, -80.9239) (157.6925, -82.0039) (158.1794, -82.9585) (158.7221, -83.7824) (159.2034, -84.3357) (159.5912, -84.691) (159.8618, -84.9014) (160, -85) knots 0 0 0 0 0 0 0.033333 0.066667 0.1 0.133333 0.166667 0.2 0.233333 0.266667 0.3 0.333333 0.366667 0.4 0.433333 0.466667 0.5 0.533333 0.566667 0.6 0.633333 0.666667 0.7 0.733333 0.766667 0.8 0.833333 0.866667 0.9 0.933333 0.966667 1 1 1 1 1 1
  line L21 (9.9467, -89.508) -> (2.9813, -89.508)
  arc A10 (238, -91.5) -> (238, -92.5) centre (238, -92) ccw
  spline S12 degree 5 poles (130, -85) (130.1382, -84.9014) (130.4088, -84.691) (130.7966, -84.3357) (131.2779, -83.7824) (131.8206, -82.9585) (132.3075, -82.0039) (132.7453, -80.9239) (133.1463, -79.7274) (133.5274, -78.4298) (133.9072, -77.0547) (134.3043, -75.6366) (134.7345, -74.223) (135.2088, -72.8764) (135.7302, -71.6789) (136.2937, -70.7262) (136.8886, -70.1082) (137.5, -69.8927) (138.1114, -70.1082) (138.7063, -70.7262) (139.2698, -71.6789) (139.7912, -72.8764) (140.2655, -74.223) (140.6957, -75.6366) (141.0928, -77.0547) (141.4726, -78.4298) (141.8537, -79.7274) (142.2547, -80.9239) (142.6925, -82.0039) (143.1794, -82.9585) (143.7221, -83.7824) (144.2034, -84.3357) (144.5912, -84.691) (144.8618, -84.9014) (145, -85) knots 0 0 0 0 0 0 0.033333 0.066667 0.1 0.133333 0.166667 0.2 0.233333 0.266667 0.3 0.333333 0.366667 0.4 0.433333 0.466667 0.5 0.533333 0.566667 0.6 0.633333 0.666667 0.7 0.733333 0.766667 0.8 0.833333 0.866667 0.9 0.933333 0.966667 1 1 1 1 1 1
  line L22 (250, -95) -> (252.5, -92.5)
  arc A11 (244.9466, -90.4891) -> (250.0533, -90.4891) centre (247.5, -89.9985) ccw
  spline S13 degree 5 poles (160, -85) (160.1382, -84.9014) (160.4088, -84.691) (160.7966, -84.3357) (161.2779, -83.7824) (161.8206, -82.9585) (162.3075, -82.0039) (162.7453, -80.9239) (163.1463, -79.7274) (163.5274, -78.4298) (163.9072, -77.0547) (164.3043, -75.6366) (164.7345, -74.223) (165.2088, -72.8764) (165.7302, -71.6789) (166.2937, -70.7262) (166.8886, -70.1082) (167.5, -69.8927) (168.1114, -70.1082) (168.7063, -70.7262) (169.2698, -71.6789) (169.7912, -72.8764) (170.2655, -74.223) (170.6957, -75.6366) (171.0928, -77.0547) (171.4726, -78.4298) (171.8537, -79.7274) (172.2547, -80.9239) (172.6925, -82.0039) (173.1794, -82.9585) (173.7221, -83.7824) (174.2034, -84.3357) (174.5912, -84.691) (174.8618, -84.9014) (175, -85) knots 0 0 0 0 0 0 0.033333 0.066667 0.1 0.133333 0.166667 0.2 0.233333 0.266667 0.3 0.333333 0.366667 0.4 0.433333 0.466667 0.5 0.533333 0.566667 0.6 0.633333 0.666667 0.7 0.733333 0.766667 0.8 0.833333 0.866667 0.9 0.933333 0.966667 1 1 1 1 1 1
  line L23 (242.5, -91.5) -> (238, -91.5)
  line L24 (244.9467, -89.508) -> (237.9813, -89.508)
  spline S14 degree 5 poles (175, -85) (175.1382, -84.9014) (175.4088, -84.691) (175.7966, -84.3357) (176.2779, -83.7824) (176.8206, -82.9585) (177.3075, -82.0039) (177.7453, -80.9239) (178.1463, -79.7274) (178.5274, -78.4298) (178.9072, -77.0547) (179.3043, -75.6366) (179.7345, -74.223) (180.2088, -72.8764) (180.7302, -71.6789) (181.2937, -70.7262) (181.8886, -70.1082) (182.5, -69.8927) (183.1114, -70.1082) (183.7063, -70.7262) (184.2698, -71.6789) (184.7912, -72.8764) (185.2655, -74.223) (185.6957, -75.6366) (186.0928, -77.0547) (186.4726, -78.4298) (186.8537, -79.7274) (187.2547, -80.9239) (187.6925, -82.0039) (188.1794, -82.9585) (188.7221, -83.7824) (189.2034, -84.3357) (189.5912, -84.691) (189.8618, -84.9014) (190, -85) knots 0 0 0 0 0 0 0.033333 0.066667 0.1 0.133333 0.166667 0.2 0.233333 0.266667 0.3 0.333333 0.366667 0.4 0.433333 0.466667 0.5 0.533333 0.566667 0.6 0.633333 0.666667 0.7 0.733333 0.766667 0.8 0.833333 0.866667 0.9 0.933333 0.966667 1 1 1 1 1 1
  line L25 (238, -92.5) -> (242.5, -92.5)
  spline S15 degree 5 poles (100, -85) (100.1382, -84.9014) (100.4088, -84.691) (100.7966, -84.3357) (101.2779, -83.7824) (101.8206, -82.9585) (102.3075, -82.0039) (102.7453, -80.9239) (103.1463, -79.7274) (103.5274, -78.4298) (103.9072, -77.0547) (104.3043, -75.6366) (104.7345, -74.223) (105.2088, -72.8764) (105.7302, -71.6789) (106.2937, -70.7262) (106.8886, -70.1082) (107.5, -69.8927) (108.1114, -70.1082) (108.7063, -70.7262) (109.2698, -71.6789) (109.7912, -72.8764) (110.2655, -74.223) (110.6957, -75.6366) (111.0928, -77.0547) (111.4726, -78.4298) (111.8537, -79.7274) (112.2547, -80.9239) (112.6925, -82.0039) (113.1794, -82.9585) (113.7221, -83.7824) (114.2034, -84.3357) (114.5912, -84.691) (114.8618, -84.9014) (115, -85) knots 0 0 0 0 0 0 0.033333 0.066667 0.1 0.133333 0.166667 0.2 0.233333 0.266667 0.3 0.333333 0.366667 0.4 0.433333 0.466667 0.5 0.533333 0.566667 0.6 0.633333 0.666667 0.7 0.733333 0.766667 0.8 0.833333 0.866667 0.9 0.933333 0.966667 1 1 1 1 1 1
  line L26 (252.5, -92.5) -> (257, -92.5)
  line L27 (250.0533, -90.4891) -> (257.0187, -90.4891)
  arc A12 (0.0354, -88.5224) -> (5.5, -97) centre (5.5, -91) ccw
  line L28 (17.5, -92.5) -> (22, -92.5)
  arc A13 (9.9466, -90.4891) -> (15.0533, -90.4891) centre (12.5, -89.9985) ccw
  spline S16 degree 5 poles (2.5, -70) (2.5, -70) (2.622, -70) (2.866, -70.0421) (3.2304, -70.2318) (3.7063, -70.7262) (4.2698, -71.6789) (4.7912, -72.8764) (5.2655, -74.223) (5.6957, -75.6366) (6.0928, -77.0547) (6.4726, -78.4298) (6.8537, -79.7274) (7.2547, -80.9239) (7.6925, -82.0039) (8.1794, -82.9585) (8.7221, -83.7824) (9.2034, -84.3357) (9.5912, -84.691) (9.8618, -84.9014) (10, -85) knots 0.5 0.5 0.5 0.5 0.5 0.5 0.5 0.533333 0.566667 0.6 0.633333 0.666667 0.7 0.733333 0.766667 0.8 0.833333 0.866667 0.9 0.933333 0.966667 1 1 1 1 1 1
  spline S17 degree 5 poles (250, -85) (250.1382, -84.9014) (250.4088, -84.691) (250.7966, -84.3357) (251.2779, -83.7824) (251.8206, -82.9585) (252.3075, -82.0039) (252.7453, -80.9239) (253.1463, -79.7274) (253.5274, -78.4298) (253.9072, -77.0547) (254.3043, -75.6366) (254.7345, -74.223) (255.2088, -72.8764) (255.7302, -71.6789) (256.2937, -70.7262) (256.7696, -70.2318) (257.134, -70.0421) (257.378, -70) (257.5, -70) (257.5, -70) knots 0 0 0 0 0 0 0.033333 0.066667 0.1 0.133333 0.166667 0.2 0.233333 0.266667 0.3 0.333333 0.366667 0.4 0.433333 0.466667 0.5 0.5 0.5 0.5 0.5 0.5 0.5
  line L29 (256.5683, -70) -> (258.4317, -70)
  arc A14 (257.5, -70) -> (260.1618, -89.0141) centre (326.7422, -70) ccw
  arc A15 (0.0354, -88.5224) -> (2.5, -70) centre (-93.3503, -66.6714) ccw
  point P0 (30, -73.5)
  point P1 (27.5, -81.5)
  point P2 (32.5, -70)
  point P3 (-2.5, -100)
  point P4 (60, -73.5)
  point P5 (57.5, -81.5)
  point P6 (35, -73.5)
  point P7 (37.5, -81.5)
  point P8 (19.5, -91)
  point P9 (65, -73.5)
  point P10 (67.5, -81.5)
  point P11 (112.5, -81.5)
  point P12 (42.5, -81.5)
  point P13 (47.5, -70)
  point P14 (50, -73.5)
  point P15 (45, -73.5)
  point P16 (52.5, -81.5)
  point P17 (62.5, -70)
  point P18 (127.5, -81.5)
  point P19 (125, -73.5)
  point P20 (122.5, -70)
  point P21 (105, -73.5)
  point P22 (120, -73.5)
  point P23 (167.5, -70)
  point P24 (102.5, -81.5)
  point P25 (87.5, -81.5)
  point P26 (110, -73.5)
  point P27 (90, -73.5)
  point P28 (82.5, -81.5)
  point P29 (170, -73.5)
  point P30 (177.5, -81.5)
  point P31 (80, -73.5)
  point P32 (107.5, -70)
  point P33 (97.5, -81.5)
  point P34 (95, -73.5)
  point P35 (180, -73.5)
  point P36 (247.5, -89.9985)
  point P37 (117.5, -81.5)
  point P38 (255, -73.5)
  point P39 (252.5, -81.5)
  point P40 (12.5, -89.9985)
  point P41 (92.5, -70)
  point P42 (222.5, -81.5)
  point P43 (227.5, -70)
  point P44 (165, -73.5)
  point P45 (185, -73.5)
  point P46 (182.5, -70)
  point P47 (187.5, -81.5)
  point P48 (192.5, -81.5)
  point P49 (195, -73.5)
  point P50 (162.5, -81.5)
  point P51 (212.5, -70)
  point P52 (15, -73.5)
  point P53 (17.5, -70)
  point P54 (20, -73.5)
  point P55 (22.5, -81.5)
  point P56 (12.5, -81.5)
  point P57 (200, -73.5)
  point P58 (197.5, -70)
  point P59 (150, -73.5)
  point P60 (202.5, -81.5)
  point P61 (147.5, -81.5)
  point P62 (155, -73.5)
  point P63 (157.5, -81.5)
  point P64 (152.5, -70)
  point P65 (242.5, -70)
  point P66 (72.5, -81.5)
  point P67 (230, -73.5)
  point P68 (75, -73.5)
  point P69 (77.5, -70)
  point P70 (140, -73.5)
  point P71 (172.5, -81.5)
  point P72 (240, -73.5)
  point P73 (247.5, -81.5)
  point P74 (232.5, -81.5)
  point P75 (217.5, -81.5)
  point P76 (210, -73.5)
  point P77 (207.5, -81.5)
  point P78 (245, -73.5)
  point P79 (237.5, -81.5)
  point P80 (137.5, -70)
  point P81 (225, -73.5)
  point P82 (132.5, -81.5)
  point P83 (142.5, -81.5)
  point P84 (135, -73.5)
  point P85 (215, -73.5)
  point P86 (5, -73.5)
  point P87 (7.5, -81.5)
  dimension "d28" = 5.2
  dimension "d29" = 2.6
  dimension "d30" = 5.2
  dimension "d31" = 2.6
  constraint coincident P36 A3.centre
  constraint horizontal L1
  constraint horizontal L17
  constraint parallel L17 L18
  constraint parallel L18 L19
  constraint parallel L19 L23
  constraint parallel L11 L20
  constraint parallel L5 L25
  constraint perpendicular L11 L22
  constraint parallel L25 L26
  constraint coincident L1.end A11
  constraint collinear L1 L24
  constraint collinear L17 L27
  constraint concentric A3 A11
  constraint coincident A7.end L1
  constraint coincident A7.start L27
  constraint coincident A2.start L24
  constraint coincident A2.end L17
  constraint coincident L17.start A2
  constraint coincident L24.end A2
  constraint coincident L27.end A7
  constraint coincident L1.start A7
  constraint coincident P40 A8.centre
  constraint horizontal L4
  constraint horizontal L7
  constraint parallel L7 L14
  constraint parallel L12 L14
  constraint parallel L0 L12
  constraint parallel L15 L16
  constraint parallel L6 L9
  constraint perpendicular L8 L16
  constraint parallel L9 L28
  constraint coincident L4.end A13
  constraint collinear L4 L21
  constraint collinear L7 L13
  constraint concentric A8 A13
  constraint coincident A0.end L4
  constraint coincident A0.start L13
  constraint coincident A4.start L21
  constraint coincident A4.end L7
  constraint coincident L7.start A4
  constraint coincident L21.end A4
  constraint coincident L13.end A0
  constraint coincident L4.start A0
  constraint tangent L2 A9
  constraint midpoint S17.end L29
  measures "d28" diameter of A11
  measures "d29" radius of A11
  measures "d30" diameter of A13
  measures "d31" radius of A13